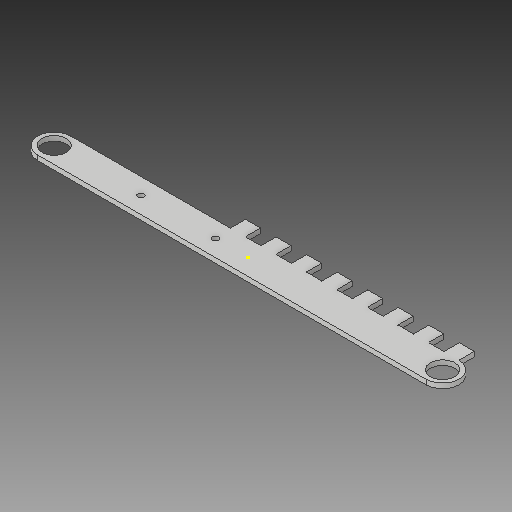
# Autodesk Inventor part: Sidewall
Saved by Autodesk Inventor 2018 (Build 220112000, 112)
## iProperties
Created: 2018-01-30
Part Number: Sidewall
Material: Generic
Document SubType Name: Modeling
Designer: alber
Density: 1 g/cm^3
Appearance: Default
Mass: 2.48729 g
Surface Area: 37.9897 cm^2
Volume: 2.48729 cm^3
Author: alber
Autodesk Inventor part; units mm, degrees
ref_plane "YZ Plane" through (0, 0, 0) normal (1, 0, 0) x (0, 1, 0)
ref_plane "XZ Plane" through (0, 0, 0) normal (0, 1, 0) x (-1, 0, 0)
ref_plane "XY Plane" through (0, 0, 0) normal (0, 0, 1) x (1, 0, 0)
sketch "Sketch1" plane through (0, 0, 0) normal (0, 1, 0) x (-1, 0, 0)
  line L0 (69, 5.4) -> (-69, 5.4)
  line L1 (-69, 5.4) -> (-69, -5.4)
  line L2 (-69, -5.4) -> (69, -5.4)
  line L3 (69, -5.4) -> (69, 5.4)
  line L4 (69, 5.4) -> (-69, -5.4) construction
  line L5 (-69, 5.4) -> (69, -5.4) construction
  point P0 (0, 0)
  dimension "d0" = 138
  dimension "d1" = 10.8
  constraints: 12 end point, 2 midpoint, 2 parallel, 1 horizontal, 1 perpendicular
  measures "d0" distance of L1.end L2.end
  measures "d1" distance of L2.end L0.start
extrude "Extrusion1" add sketch "Sketch1" along normal blind 1.6
sketch "Sketch2" plane through (0, 1.6, 0) normal (0, 1, 0) x (1, 0, 0)
  line L0 (-96.6, 0) -> (96.6, 0) projected
  circle A0 centre (-35.2, 0) radius 1
  circle A1 centre (-10.8, 0) radius 1
  line L1 (-69, 5.4) -> (-69, -5.4) projected
  point P0 (0, 0)
  dimension "d4" = 58.2
  dimension "d5" = 33.8
  dimension "d6" = 2
  constraints: 2 centre point, 2 point on line, 1 equal radius
  measures "d4" distance from line of L1 A1.centre
  measures "d5" distance from line of L1 A0.centre
  measures "d6" diameter of A0
extrude "Extrusion2" cut sketch "Sketch2" against normal through all
sketch "Sketch3" plane through (0, 1.6, 0) normal (0, 1, 0) x (1, 0, 0)
  line L0 (-96.6, 0) -> (96.6, 0) projected
  circle A0 centre (-63.6, 0) radius 4
  line L1 (-69, 5.4) -> (-69, -5.4) projected
  point P0 (0, 0)
  dimension "d9" = 5.4
  dimension "d10" = 8
  constraints: 1 centre point, 1 point on line
  measures "d9" distance from line of L1 A0.centre
  measures "d10" diameter of A0
extrude "Extrusion3" cut sketch "Sketch3" against normal through all
full round fillet "Fillet1" first side at (-23, 1.0667, 5.4) centre faces at (-69, 0.5333, -1.8) second side at (23, 1.0667, -5.4)
mirror "Mirror1" about plane through (0, 0, 0) normal (1, 0, 0) of "Extrusion3", "Fillet1"
sketch "Sketch4" plane through (0, 1.6, 0) normal (0, 1, 0) x (1, 0, 0)
  point P0 (0, 0)
sketch "Sketch5" plane through (0, 1.6, 0) normal (0, 1, 0) x (1, 0, 0)
  line L0 (63.6, 5.4) -> (58.7, 5.4)
  line L1 (58.7, 5.4) -> (58.7, 10.4)
  line L2 (58.7, 10.4) -> (63.6, 10.4)
  line L3 (63.6, 10.4) -> (63.6, 5.4)
  point P0 (0, 0)
  dimension "d13" = 5
  dimension "d14" = 4.9
  constraints: 8 end point, 2 parallel, 1 horizontal, 1 perpendicular
  measures "d13" distance of L2.end L0.start
  measures "d14" distance of L1.end L2.end
extrude "Extrusion4" add sketch "Sketch5" against normal up to surface (1.6 mm away)
pattern_linear "Rectangular Pattern1" count 8 spacing 10 along (-1, 0, 0) of "Extrusion4"
sketch "Sketch6" plane through (0, 0, 0) normal (0, -1, 0) x (1, 0, 0)
  arc A0 (63.6, -5.4) -> (63.6, 5.4) centre (63.6, 0) ccw projected
  line L0 (-63.6, 5.4) -> (63.6, 5.4) projected
  arc A1 (-63.6, 5.4) -> (-63.6, -5.4) centre (-63.6, 0) ccw projected
  line L1 (-11.3, -5.4) -> (-63.6, -5.4) projected
  line L2 (-11.3, -5.4) -> (-11.3, -10.4) projected
  line L3 (-11.3, -10.4) -> (-6.4, -10.4) projected
  line L4 (-6.4, -10.4) -> (-6.4, -5.4) projected
  line L5 (-1.3, -5.4) -> (-6.4, -5.4) projected
  line L6 (-1.3, -5.4) -> (-1.3, -10.4) projected
  line L7 (-1.3, -10.4) -> (3.6, -10.4) projected
  line L8 (3.6, -10.4) -> (3.6, -5.4) projected
  line L9 (8.7, -5.4) -> (3.6, -5.4) projected
  line L10 (8.7, -5.4) -> (8.7, -10.4) projected
  line L11 (8.7, -10.4) -> (13.6, -10.4) projected
  line L12 (13.6, -10.4) -> (13.6, -5.4) projected
  line L13 (18.7, -5.4) -> (13.6, -5.4) projected
  line L14 (18.7, -5.4) -> (18.7, -10.4) projected
  line L15 (18.7, -10.4) -> (23.6, -10.4) projected
  line L16 (23.6, -10.4) -> (23.6, -5.4) projected
  line L17 (28.7, -5.4) -> (23.6, -5.4) projected
  line L18 (28.7, -5.4) -> (28.7, -10.4) projected
  line L19 (28.7, -10.4) -> (33.6, -10.4) projected
  line L20 (33.6, -10.4) -> (33.6, -5.4) projected
  line L21 (38.7, -5.4) -> (33.6, -5.4) projected
  line L22 (38.7, -5.4) -> (38.7, -10.4) projected
  line L23 (38.7, -10.4) -> (43.6, -10.4) projected
  line L24 (43.6, -10.4) -> (43.6, -5.4) projected
  line L25 (48.7, -5.4) -> (43.6, -5.4) projected
  line L26 (48.7, -5.4) -> (48.7, -10.4) projected
  line L27 (48.7, -10.4) -> (53.6, -10.4) projected
  line L28 (53.6, -10.4) -> (53.6, -5.4) projected
  line L29 (58.7, -5.4) -> (53.6, -5.4) projected
  line L30 (58.7, -5.4) -> (58.7, -10.4) projected
  line L31 (58.7, -10.4) -> (63.6, -10.4) projected
  line L32 (63.6, -10.4) -> (63.6, -5.4) projected
  circle A2 centre (63.6, 0) radius 4 projected
  circle A3 centre (-63.6, 0) radius 4 projected
  circle A4 centre (-35.2, 0) radius 1 projected
  circle A5 centre (-10.8, 0) radius 1 projected
  arc A6 (63.6, -15) -> (49.6057, 5.4) centre (63.6, 0) ccw
  circle A7 centre (-63.6, 0) radius 4 projected
  arc A8 (-49.6057, 5.4) -> (-49.6057, -5.4) centre (-63.6, 0) ccw
  line L33 (63.6, -10.4) -> (63.6, -15)
  point P0 (0, 0)
  dimension "d20" = 30
  dimension "d21" = 30
  constraints: 4 point on circle, 3 point on line, 2 centre point, 2 coincident, 2 end point
  measures "d20" diameter of A6
  measures "d21" diameter of A8
extrude "Extrusion5" [suppressed]
body "Solid1"
